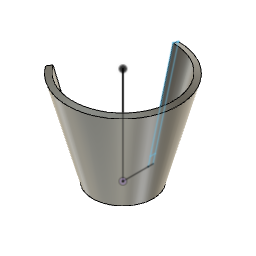
LED Shield v2 (Autodesk Fusion 360 design; units mm, degrees)
Autodesk Fusion 360 part; units mm, degrees
sketch "Sketch1" plane through (0, 0, 0) normal (1, 0, 0) x (0, 1, 0)
  line L0 (0, 0) -> (0, 10)
  line L1 (0, 0) -> (2.6, 0)
  line L2 (2.6, 0) -> (3.1, 0)
  line L3 (3.1, 0) -> (5.6976, 9.57)
  line L4 (5.6976, 9.57) -> (5.1602, 9.7159)
  line L5 (5.1602, 9.7159) -> (2.6, 0)
  line L6 (2.814, 0.8123) -> (3.3205, 0.8123)
  dimension "d1" = 10
  dimension "d2" = 2.6
  dimension "d3" = 0.5
  constraint coincident L0.start L1.start
  constraint vertical L0
  constraint perpendicular L0 L1
  constraint parallel L1 L2
  constraint perpendicular L3 L4
  constraint coincident L5 L6.start
  constraint coincident L3 L6.end
  constraint horizontal L6
  measures "d1" distance of L0.start L0.end
  measures "d2" distance of L0.start L1.end
  measures "d3" distance of L1.end L2.end
revolve "Revolve1" add sketch "Sketch1" angle 235 about axis through (0, 0, 0) along (0, 0, -1) contours L3 L4 L5 L6
revolve "Revolve2" add sketch "Sketch1" angle 360 about axis through (0, 0, 0) along (0, 0, 1) contours L2 L3 L5 L6
